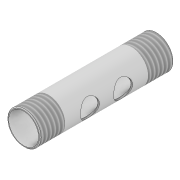
# Autodesk Inventor part: Wasserverteiler1
Saved by Autodesk Inventor 2021 (Build 250183000, 183)
## iProperties
Created: 2021-10-22
Part Number: Wasserverteiler1
Material: Generisch
Document SubType Name: Modeling
Designer: lukas
Density: 1 g/cm^3
Appearance: Vorgabe
Author: lukas
Autodesk Inventor part; units mm, degrees
ref_plane "XZ Plane" through (0, 0, 0) normal (0, 1, 0) x (-1, 0, 0)
ref_plane "XY Plane" through (0, 0, 0) normal (0, 0, 1) x (1, 0, 0)
sketch "Skizze1" plane through (0, 0, 0) normal (0, 0, 1) x (1, 0, 0)
  line L0 (-14, 0) -> (14, 0) projected
  line L1 (0, -14) -> (0, 14) projected
  circle A0 centre (0, 0) radius 10
  circle A1 centre (0, 0) radius 9
  dimension "d0" = 20
  dimension "d1" = 18
  constraints: 2 centre point, 2 coincident
  measures "d0" diameter of A0
  measures "d1" diameter of A1
extrude "Extrusion1" add sketch "Skizze1" along normal blind 80 contours A1 L1 A0 L0 | L0 A0 L1 A1 | A1 L0 A0 L1 | L1 A0 L0 A1
thread "Gewinde1" size "M20x2.5" class "6g" standard "ANSI Metric M Profile" length 15
thread "Gewinde2" size "M20x2.5" class "6g" standard "ANSI Metric M Profile" length 15
chamfer "Fase1" distance 0.5 angle 45 1 edges at (-10, 0, 80)
ref_plane "Arbeitsebene1" through (10, 0, 0) normal (1, 0, 0) x (0, 1, 0)
sketch "Skizze2" plane through (10, 0, 0) normal (1, 0, 0) x (0, 1, 0)
  line L0 (-9.5, 80) -> (9.5, 80) projected
  point P0 (0, 0)
  point P1 (0, 50)
  point P2 (0, 30)
  dimension "d12" = 30
  dimension "d13" = 30
  measures "d12" distance of point (0, 0) point (0, 30)
  measures "d13" distance from line of point (0, 50) L0
hole "Bohrung1" at (10, 0, 50) at (10, 0, 30) direction (-1, 0, 0) diameter 11.445 end through all thread size "G13.157x1.337" designation "G 1/4" standard "ISO Pipe Threads"
